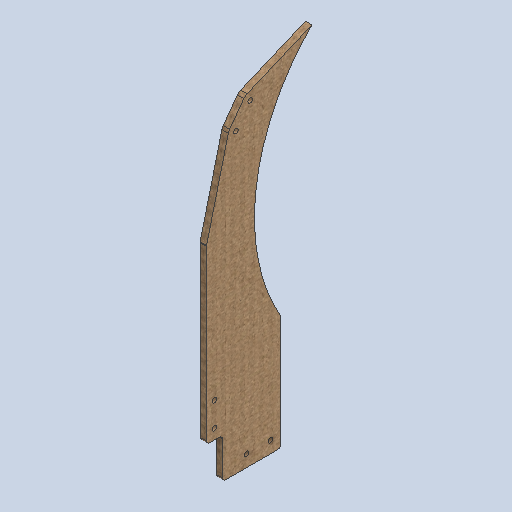
# Autodesk Inventor part: hand-grab-v1-Plate-arm
Saved by Autodesk Inventor 2025.1 (Build 291241000, 241)
## iProperties
Created: 2024-10-12
Part Number: hand-grab-v1-Plate-arm
Material: MDF 中密度繊維ボード
Document SubType Name: Modeling
Designer: haruy
Density: 0.8 g/cm^3
Appearance: ダンボール - 段ボール紙
Author: haruy
Autodesk Inventor part; units mm, degrees
ref_plane "YZ Plane" through (0, 0, 0) normal (1, 0, 0) x (0, 1, 0)
ref_plane "XZ Plane" through (0, 0, 0) normal (0, 1, 0) x (-1, 0, 0)
ref_plane "XY Plane" through (0, 0, 0) normal (0, 0, 1) x (1, 0, 0)
derived "hand-grab-v2-Sketch-Base.ipt"
sketch "スケッチ1" plane through (300, 0, 0) normal (1, 0, 0) x (0, 1, 0)
  circle A0 centre (0, 0) radius 122.5
  line L0 (-136.5, 142.5) -> (-132.5, 142.5)
  line L1 (-132.5, 142.5) -> (-132.5, -206.7109)
  line L2 (-132.5, -206.7109) -> (-136.5, -206.7109)
  line L3 (-136.5, -206.7109) -> (-136.5, 142.5)
  line L4 (0, 0) -> (86.6206, 86.6206)
  line L5 (0, 0) -> (0, 122.5)
  line L6 (0, 0) -> (-61.25, 106.0881)
  line L7 (-150.5, 12.2) -> (-198.3, 12.2)
  line L8 (-198.3, 12.2) -> (-198.3, -12.2)
  line L9 (-198.3, -12.2) -> (-150.5, -12.2)
  line L10 (-150.5, -12.2) -> (-150.5, 12.2)
  line L11 (-150.5, 6.5) -> (-147.9, 6.5)
  line L12 (-147.9, 6.5) -> (-147.9, -6.5)
  line L13 (-147.9, -6.5) -> (-150.5, -6.5)
  line L14 (-150.5, -6.5) -> (-150.5, 6.5)
  line L15 (-147.9, 3) -> (-133.5, 3)
  line L16 (-133.5, 3) -> (-133.5, -3)
  line L17 (-133.5, -3) -> (-147.9, -3)
  line L18 (-147.9, -3) -> (-147.9, 3)
  line L19 (-146.5, 70.3296) -> (-150.5, 70.3296)
  line L20 (-150.5, 70.3296) -> (-150.5, -72.1331)
  line L21 (-150.5, -72.1331) -> (-146.5, -72.1331)
  line L22 (-146.5, -72.1331) -> (-146.5, 70.3296)
  line L23 (-136.5, 9) -> (-142.5, 9)
  line L24 (-142.5, 9) -> (-142.5, -9)
  line L25 (-142.5, -9) -> (-136.5, -9)
  line L26 (-136.5, -9) -> (-136.5, 9)
  line L27 (-61.25, 106.0881) -> (-132.5, 106.0881)
  circle A1 centre (-532.5, 0) radius 600
  line L28 (-132.5, 142.5) -> (-7.6064, 142.5)
  arc A2 (86.6206, 86.6206) -> (-7.6064, 142.5) centre (3, 53) ccw
  circle A3 centre (-532.5, 0) radius 400
  circle A4 centre (-134, 133.5) radius 1.5
  circle A5 centre (-134, 115.5) radius 1.5
  line L29 (-132.5, 106.0881) -> (-136.5, 106.0881)
  line L30 (-132.5, 142.5) -> (-117.5, 142.5)
  line L31 (-117.5, 142.5) -> (-117.5, 106.0881)
  line L32 (-117.5, 106.0881) -> (-132.5, 106.0881)
  line L33 (-132.5, 106.0881) -> (-132.5, 142.5)
  circle A6 centre (-125, 127.5) radius 1.5
  circle A7 centre (-125, 112.5) radius 1.5
  line L34 (-107.5, 142.5) -> (-107.5, 106.0881)
  circle A8 centre (65, 125.1457) radius 1.5
  circle A9 centre (-86, 147.5) radius 1.5
  circle A10 centre (65, 125.1457) radius 5
  circle A11 centre (-86, 147.5) radius 5
  line L35 (-91, 147.5) -> (-91, 142.5)
  line L36 (-81, 147.5) -> (-81, 142.5)
  circle A12 centre (-101, 147.5) radius 5
  circle A13 centre (-101, 147.5) radius 1.5
  line L37 (-107.5, 142.5) -> (-107.5, 152.5)
  line L38 (-107.5, 152.5) -> (0, 152.5)
  circle A14 centre (52.8883, 133.9948) radius 5
  circle A15 centre (52.8883, 133.9948) radius 1.5
  circle A16 centre (-332.5, 0) radius 600
  line L39 (86.6206, 86.6206) -> (69.6092, 127.0835)
  line L40 (0, 152.5) -> (54.1119, 138.8428)
  line L41 (55.838, 138.0321) -> (67.9497, 129.183)
  point P0 (-132.5, 124.2941)
  point P1 (60.8327, 127.9086)
  point P2 (16.7537, 142.0706)
  point P3 (60.7909, 127.8445)
  point P4 (26.7893, 139.9299)
  point P5 (60.8975, 128.0039)
  point P6 (60.9197, 128.0355)
  point P7 (-86, 152.5)
  point P8 (-86, 142.5)
  point P9 (61.7412, 121.3536)
  dimension "d1" = 3
  dimension "d2" = 3
  dimension "d3" = 9
  dimension "d4" = 18
  dimension "d5" = 2.5
  dimension "d6" = 2.5
  dimension "d9" = 15
  dimension "d10" = 0
  dimension "d11" = 3
  dimension "d12" = 3
  dimension "d13" = 15
  dimension "d14" = 15
  dimension "d15" = 7.5
  dimension "d16" = 7.5
  dimension "d22" = 10
  dimension "d27" = 3
  dimension "d28" = 3
  dimension "d29" = 10
  dimension "d30" = 10
  dimension "d32" = 86
  dimension "d33" = 10
  dimension "d34" = 3
  dimension "d35" = 15
  dimension "d36" = 10
  dimension "d37" = 3
  dimension "d38" = 15
  dimension "d40" = 65
  measures "d1" diameter of A4
  measures "d2" diameter of A5
  measures "d3" distance from line of A4.centre L0
  measures "d4" distance of A5.centre A4.centre
  measures "d5" distance from line of A4.centre L3
  measures "d6" distance from line of A5.centre L3
  measures "d9" distance of L31.end L32.end
  measures "d10" distance between parallel lines of L27 L32
  measures "d11" diameter of A6
  measures "d12" diameter of A7
  measures "d13" distance from line of L30 A6.centre
  measures "d14" distance of A7.centre A6.centre
  measures "d15" distance from line of A7.centre L1
  measures "d16" horizontal distance of A6.centre point (-132.5, 124.294)
  measures "d22" distance between parallel lines of L31 L34
  measures "d27" diameter of A8
  measures "d28" diameter of A9
  measures "d29" diameter of A10
  measures "d30" diameter of A11
  measures "d32" horizontal distance of point (0, 0) A11.centre
  measures "d33" diameter of A12
  measures "d34" diameter of A13
  measures "d35" distance of A12.centre A9.centre
  measures "d36" diameter of A14
  measures "d37" diameter of A15
  measures "d38" distance of A14.centre A8.centre
  measures "d40" horizontal distance of point (0, 0) A8.centre
sketch "スケッチ2" plane through (0, -300, 0) normal (0, 1, 0) x (-1, 0, 0)
  circle A0 centre (0, 0) radius 122.5
  line L0 (-34, 142.5) -> (-30, 142.5)
  line L1 (-30, 142.5) -> (-30, 106)
  line L2 (-30, 106) -> (-34, 106)
  line L3 (-34, 106) -> (-34, 142.5)
  line L4 (30, 142.5) -> (34, 142.5)
  line L5 (34, 142.5) -> (34, 106)
  line L6 (34, 106) -> (30, 106)
  line L7 (30, 106) -> (30, 142.5)
  circle A1 centre (0, 0) radius 12.5
  line L8 (-30, 142.5) -> (30, 142.5)
  line L9 (-12.5, 103.9737) -> (-12.5, -60)
  line L10 (-12.5, -60) -> (-30, -60)
  line L11 (-30, -60) -> (-30, 142.5)
  line L12 (-30, 142.5) -> (-12.5, 142.5)
  line L13 (-12.5, 142.5) -> (-12.5, -60)
  line L14 (-30, 20) -> (-12.5, 20)
  line L15 (-4.5, 136) -> (4.5, 136)
  line L16 (4.5, 136) -> (4.5, 41)
  line L17 (4.5, 41) -> (-4.5, 41)
  line L18 (-4.5, 41) -> (-4.5, 136)
  line L19 (10, 128.5) -> (-10, 128.5)
  line L20 (-10, 128.5) -> (-10, 98.5)
  line L21 (-10, 98.5) -> (10, 98.5)
  line L22 (10, 98.5) -> (10, 128.5)
  line L23 (-12.5, 20) -> (-11.5, 20)
  line L24 (-11.5, 20) -> (-11.5, -60)
  line L25 (-11.5, -60) -> (-12.5, -60)
  line L26 (-12.5, -60) -> (-12.5, 20)
  line L27 (-11.5, 20) -> (-13.8, 19.214)
  line L28 (-13.8, 19.214) -> (-13.8, 18.429)
  line L29 (-13.8, 18.429) -> (-11.5, 17.643)
  line L30 (-11.5, 17.643) -> (-11.5, 20)
  line L31 (-11.5, 16.8584) -> (-13.8, 16.0724)
  line L32 (-13.8, 15.2874) -> (-11.5, 14.5014)
  line L33 (-13.8, 16.0724) -> (-13.8, 15.2874)
  line L34 (-11.5, 13.7168) -> (-13.8, 12.9308)
  line L35 (-13.8, 12.1458) -> (-11.5, 11.3598)
  line L36 (-13.8, 12.9308) -> (-13.8, 12.1458)
  line L37 (-11.5, 10.5752) -> (-13.8, 9.7892)
  line L38 (-13.8, 9.0042) -> (-11.5, 8.2182)
  line L39 (-13.8, 9.7892) -> (-13.8, 9.0042)
  line L40 (-11.5, 7.4336) -> (-13.8, 6.6476)
  line L41 (-13.8, 5.8626) -> (-11.5, 5.0766)
  line L42 (-13.8, 6.6476) -> (-13.8, 5.8626)
  line L43 (-11.5, 4.292) -> (-13.8, 3.506)
  line L44 (-13.8, 2.721) -> (-11.5, 1.935)
  line L45 (-13.8, 3.506) -> (-13.8, 2.721)
  line L46 (-11.5, 1.1505) -> (-13.8, 0.3645)
  line L47 (-13.8, -0.4205) -> (-11.5, -1.2065)
  line L48 (-13.8, 0.3645) -> (-13.8, -0.4205)
  line L49 (-11.5, -1.9911) -> (-13.8, -2.7771)
  line L50 (-13.8, -3.5621) -> (-11.5, -4.3481)
  line L51 (-13.8, -2.7771) -> (-13.8, -3.5621)
  line L52 (-11.5, -5.1327) -> (-13.8, -5.9187)
  line L53 (-13.8, -6.7037) -> (-11.5, -7.4897)
  line L54 (-13.8, -5.9187) -> (-13.8, -6.7037)
  line L55 (-11.5, -8.2743) -> (-13.8, -9.0603)
  line L56 (-13.8, -9.8453) -> (-11.5, -10.6313)
  line L57 (-13.8, -9.0603) -> (-13.8, -9.8453)
  line L58 (-11.5, -11.4159) -> (-13.8, -12.2019)
  line L59 (-13.8, -12.9869) -> (-11.5, -13.7729)
  line L60 (-13.8, -12.2019) -> (-13.8, -12.9869)
  line L61 (-11.5, -14.5575) -> (-13.8, -15.3435)
  line L62 (-13.8, -16.1285) -> (-11.5, -16.9145)
  line L63 (-13.8, -15.3435) -> (-13.8, -16.1285)
  line L64 (-11.5, -17.6991) -> (-13.8, -18.4851)
  line L65 (-13.8, -19.2701) -> (-11.5, -20.0561)
  line L66 (-13.8, -18.4851) -> (-13.8, -19.2701)
  line L67 (-11.5, -20.8407) -> (-13.8, -21.6267)
  line L68 (-13.8, -22.4117) -> (-11.5, -23.1977)
  line L69 (-13.8, -21.6267) -> (-13.8, -22.4117)
  line L70 (-11.5, -23.9823) -> (-13.8, -24.7683)
  line L71 (-13.8, -25.5533) -> (-11.5, -26.3393)
  line L72 (-13.8, -24.7683) -> (-13.8, -25.5533)
  line L73 (-11.5, -27.1238) -> (-13.8, -27.9099)
  line L74 (-13.8, -28.6949) -> (-11.5, -29.4809)
  line L75 (-13.8, -27.9099) -> (-13.8, -28.6949)
  line L76 (-11.5, -30.2654) -> (-13.8, -31.0514)
  line L77 (-13.8, -31.8364) -> (-11.5, -32.6224)
  line L78 (-13.8, -31.0514) -> (-13.8, -31.8364)
  line L79 (-11.5, -33.407) -> (-13.8, -34.193)
  line L80 (-13.8, -34.978) -> (-11.5, -35.764)
  line L81 (-13.8, -34.193) -> (-13.8, -34.978)
  line L82 (-11.5, -36.5486) -> (-13.8, -37.3346)
  line L83 (-13.8, -38.1196) -> (-11.5, -38.9056)
  line L84 (-13.8, -37.3346) -> (-13.8, -38.1196)
  line L85 (-11.5, -39.6902) -> (-13.8, -40.4762)
  line L86 (-13.8, -41.2612) -> (-11.5, -42.0472)
  line L87 (-13.8, -40.4762) -> (-13.8, -41.2612)
  line L88 (-11.5, -42.8318) -> (-13.8, -43.6178)
  line L89 (-13.8, -44.4028) -> (-11.5, -45.1888)
  line L90 (-13.8, -43.6178) -> (-13.8, -44.4028)
  line L91 (-11.5, -45.9734) -> (-13.8, -46.7594)
  line L92 (-13.8, -47.5444) -> (-11.5, -48.3304)
  line L93 (-13.8, -46.7594) -> (-13.8, -47.5444)
  line L94 (-11.5, -49.115) -> (-13.8, -49.901)
  line L95 (-13.8, -50.686) -> (-11.5, -51.472)
  line L96 (-13.8, -49.901) -> (-13.8, -50.686)
  line L97 (-11.5, -52.2566) -> (-13.8, -53.0426)
  line L98 (-13.8, -53.8276) -> (-11.5, -54.6136)
  line L99 (-13.8, -53.0426) -> (-13.8, -53.8276)
  line L100 (-11.5, -55.3982) -> (-13.8, -56.1842)
  line L101 (-13.8, -56.9692) -> (-11.5, -57.7552)
  line L102 (-13.8, -56.1842) -> (-13.8, -56.9692)
  line L103 (-11.5, -58.5397) -> (-13.8, -59.3258)
  line L104 (-13.8, -60.1108) -> (-11.5, -60.8968)
  line L105 (-13.8, -59.3258) -> (-13.8, -60.1108)
  line L106 (-13.8, 20) -> (-13.8, -60)
  line L107 (-13.8, -59.3258) -> (-30, -59.3258)
  line L108 (-13.8, 18.429) -> (-30, 18.429)
  line L109 (-13.8, 18.429) -> (-13.8, 142.5)
  line L110 (-34, 137.5) -> (34, 137.5)
  line L111 (-34, 117.5) -> (34, 117.5)
  line L112 (30, 106) -> (-13.8, 106)
  line L113 (32, -142.5) -> (30, -142.5)
  line L114 (30, -142.5) -> (30, -106)
  line L115 (30, -106) -> (32, -106)
  line L116 (32, -106) -> (32, -142.5)
  line L117 (-32, -106) -> (-30, -106)
  line L118 (-30, -106) -> (-30, -142.5)
  line L119 (-30, -142.5) -> (-32, -142.5)
  line L120 (-32, -142.5) -> (-32, -106)
  line L121 (30, -142.5) -> (-30, -142.5)
  line L122 (30, -142.5) -> (12.5, -142.5)
  line L123 (12.5, -142.5) -> (12.5, 80)
  line L124 (12.5, 80) -> (30, 80)
  line L125 (30, 80) -> (30, -142.5)
  line L126 (-30, -106) -> (12.5, -106)
  line L127 (-4.5, -41) -> (4.5, -41)
  line L128 (4.5, -41) -> (4.5, -136)
  line L129 (4.5, -136) -> (-4.5, -136)
  line L130 (-4.5, -136) -> (-4.5, -41)
  line L131 (-10, -98.5) -> (10, -98.5)
  line L132 (10, -98.5) -> (10, -128.5)
  line L133 (10, -128.5) -> (-10, -128.5)
  line L134 (-10, -128.5) -> (-10, -98.5)
  line L135 (-32, 202.1278) -> (-17, 202.1278)
  line L136 (-17, 202.1278) -> (-17, -209.3238)
  line L137 (-17, -209.3238) -> (-32, -209.3238)
  line L138 (-32, -209.3238) -> (-32, 202.1278)
  line L139 (17, 202.1278) -> (32, 202.1278)
  line L140 (32, 202.1278) -> (32, -266.5661)
  line L141 (32, -266.5661) -> (17, -266.5661)
  line L142 (17, -266.5661) -> (17, 202.1278)
  line L143 (4.5, 41) -> (-13.8, 41)
  line L144 (-30, 30) -> (-12.65, 30)
  line L145 (-30, 142.5) -> (-15, 142.5)
  line L146 (-15, 142.5) -> (-15, 106)
  line L147 (-15, 106) -> (-30, 106)
  line L148 (-30, 106) -> (-30, 142.5)
  line L149 (30, 142.5) -> (15, 142.5)
  line L150 (15, 142.5) -> (15, 106)
  line L151 (15, 106) -> (30, 106)
  line L152 (30, 106) -> (30, 142.5)
  line L153 (-13.8, 21.571) -> (-11.5, 20.785)
  line L154 (-11.5, 20.0004) -> (-13.8, 19.2144)
  line L155 (-13.8, 24.713) -> (-11.5, 23.927)
  line L156 (-11.5, 23.1424) -> (-13.8, 22.3564)
  line L157 (-13.8, 27.855) -> (-11.5, 27.069)
  line L158 (-11.5, 26.2844) -> (-13.8, 25.4984)
  line L159 (-13.8, 30.997) -> (-11.5, 30.211)
  line L160 (-11.5, 29.4264) -> (-13.8, 28.6404)
  line L161 (-11.5, 20.0004) -> (-11.5, 27.069)
  line L162 (-13.8, 27.855) -> (-30, 27.855)
  point P0 (21.25, -142.5)
  point P1 (-22.5, 142.5)
ref_plane "作業平面1" through (0, -300, 0) normal (0, 1, 0) x (-1, 0, 0)
ref_plane "作業平面2" through (300, 0, 0) normal (1, 0, 0) x (0, 1, 0)
extrude "押し出し1" add sketch "スケッチ1" along normal blind 4 contours A0 A1 A2 L39 | A0 L27 L34 L28 A2 A1 | A2 A10 L39 | A2 A14 A1 | A1 A14 L41 A10 A2 | A10 | L27 L31 L28 L34 | A14 A1 A15 | A1 A15 A14 | A2 L28 L36 A11 L38 L40 A1 A14 | L27 L1 L28 L31 | L37 L38 A12 L28 | L40 A14 A1 | A12 L38 A11 L35 L28 | A12 | L28 A11 L36 | L35 A11 L28 | A11
fillet "フィレット1" radius 2 5 edges at (302, -107.5, 142.5) (302, -107.5, 152.5) (302, -132.5, 142.5) (302, -132.5, 106.0881) (302, 0, 152.5)
sketch "スケッチ3" plane through (304, -105.5, 152.5) normal (1, 0, 0) x (0, 0, -1)
  arc A0 (0.0608, 105.7409) -> (0, 105.2515) centre (2, 105.2515) ccw projected
  line L0 (0, 105.2515) -> (0, 0) projected
  arc A1 (0, 0) -> (2, -2) centre (2, 0) ccw projected
  line L1 (2, -2) -> (8, -2) projected
  arc A2 (10, -4) -> (8, -2) centre (8, -4) ccw projected
  line L2 (10, -4) -> (10, -25) projected
  arc A3 (10, -25) -> (12, -27) centre (12, -25) ccw projected
  line L3 (12, -27) -> (44.4119, -27) projected
  arc A4 (44.4119, -27) -> (46.4119, -25) centre (44.4119, -25) ccw projected
  line L4 (46.4119, -25) -> (46.4119, 44.25) projected
  arc A5 (65.8794, 192.1206) -> (46.4119, 44.25) centre (152.5, 105.5) ccw projected
  line L5 (65.8794, 192.1206) -> (25.4165, 175.1092) projected
  arc A6 (25.4165, 175.1092) -> (23.317, 173.4497) centre (27.3543, 170.5) ccw projected
  line L6 (23.317, 173.4497) -> (14.4679, 161.338) projected
  arc A7 (14.4679, 161.338) -> (13.6572, 159.6119) centre (18.5052, 158.3883) ccw projected
  line L7 (13.6572, 159.6119) -> (0.0608, 105.7409) projected
  circle A8 centre (27.3543, 170.5) radius 1.5 projected
  circle A9 centre (5, 4.5) radius 1.5 projected
  circle A10 centre (5, 19.5) radius 1.5 projected
  circle A11 centre (18.5052, 158.3883) radius 1.5 projected
  circle A12 centre (25, -19.5) radius 1.5 projected
  circle A13 centre (40, -19.5) radius 1.5 projected
equation "\"d6\" = d5"
equation "\"d16\" = d15"
